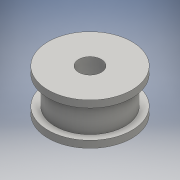
# Autodesk Inventor part: poulie v2
Saved by Autodesk Inventor 2016 (Build 200138000, 138)
## iProperties
Created: 2016-02-21
Part Number: poulie v2
Material: Generic
Document SubType Name: Modeling
Designer: Thetheos
Density: 1 g/cm^3
Appearance: Default
Mass: 3.92463 g
Surface Area: 21.6416 cm^2
Volume: 3.92463 cm^3
Author: Thetheos
Autodesk Inventor part; units mm, degrees
ref_plane "YZ Plane" through (0, 0, 0) normal (1, 0, 0) x (0, 1, 0)
ref_plane "XZ Plane" through (0, 0, 0) normal (0, 1, 0) x (-1, 0, 0)
ref_plane "XY Plane" through (0, 0, 0) normal (0, 0, 1) x (1, 0, 0)
sketch "Sketch1" plane through (0, 0, 0) normal (0, 0, 1) x (1, 0, 0)
  circle A0 centre (0, 0) radius 10
  circle A1 centre (0, 0) radius 3.25
  dimension "d0" = 20
  dimension "d1" = 6.5
  constraints: 3 coincident, 2 centre point
  measures "d0" diameter of A0
  measures "d1" diameter of A1
extrude "Extrusion1" add sketch "Sketch1" along normal blind 12
sketch "Sketch2" plane through (0, 0, 12) normal (0, 0, 1) x (1, 0, 0)
  circle A0 centre (0, 0) radius 12
  dimension "d4" = 24
  constraints: 1 centre point, 1 coincident
  measures "d4" diameter of A0
extrude "Extrusion2" add sketch "Sketch2" against normal blind 2
sketch "Sketch3" plane through (0, 0, 12) normal (0, 0, 1) x (1, 0, 0)
  circle A0 centre (0, 0) radius 3.25
  dimension "d7" = 6.5
  constraints: 1 centre point, 1 coincident
  measures "d7" diameter of A0
sketch "Sketch4" plane through (0, 0, 0) normal (0, 0, -1) x (-1, 0, 0)
  circle A0 centre (0, 0) radius 12
  circle A1 centre (0, 0) radius 10
  dimension "d8" = 24
  constraints: 2 centre point, 2 coincident
  measures "d8" diameter of A0
extrude "Extrusion3" add sketch "Sketch4" against normal blind 2
extrude "Extrusion4" cut sketch "Sketch3" against normal through all
body "Solid1"
